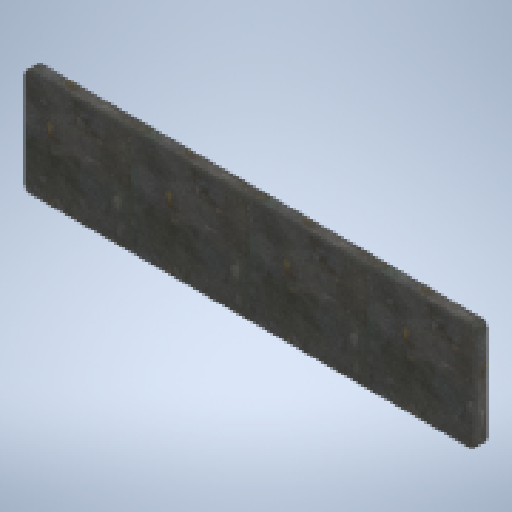
# Autodesk Inventor part: MountingPlate
Saved by Autodesk Inventor 2023 (Build 270158000, 158)
## iProperties
Created: 2023-07-27
Part Number: MountingPlate
Material: Steel
Document SubType Name: Modeling
Designer: Parker
Density: 7.85 g/cm^3
Appearance: Plate
Author: Parker
Autodesk Inventor part; units mm, degrees
ref_plane "YZ Plane" through (0, 0, 0) normal (1, 0, 0) x (0, 1, 0)
ref_plane "XZ Plane" through (0, 0, 0) normal (0, 1, 0) x (-1, 0, 0)
ref_plane "XY Plane" through (0, 0, 0) normal (0, 0, 1) x (1, 0, 0)
sketch "Sketch1" plane through (0, 0, 0) normal (0, 0, 1) x (1, 0, 0)
  circle A0 centre (323.7, 80.7) radius 3.75 projected
  circle A1 centre (224.8, -20.2) radius 3.75 projected
  line L0 (219.8, -29.2) -> (328.7, -29.2) projected
  arc A2 (215.8, -25.2) -> (219.8, -29.2) centre (219.8, -25.2) ccw projected
  line L1 (215.8, 85.7) -> (215.8, -25.2) projected
  arc A3 (219.8, 89.7) -> (215.8, 85.7) centre (219.8, 85.7) ccw projected
  line L2 (328.7, 89.7) -> (219.8, 89.7) projected
  arc A4 (332.7, 85.7) -> (328.7, 89.7) centre (328.7, 85.7) ccw projected
  line L3 (332.7, -25.2) -> (332.7, 85.7) projected
  arc A5 (328.7, -29.2) -> (332.7, -25.2) centre (328.7, -25.2) ccw projected
  circle A6 centre (224.8, 80.7) radius 3.75 projected
  circle A7 centre (323.7, -20.2) radius 3.75 projected
  circle A8 centre (-229.1, -19.7) radius 3.75 projected
  circle A9 centre (-288.2, -19.7) radius 3.75 projected
  circle A10 centre (-170, 80.7) radius 3.75 projected
  line L4 (-165, 89.7) -> (-293.2, 89.7) projected
  arc A11 (-161, 85.7) -> (-165, 89.7) centre (-165, 85.7) ccw projected
  line L5 (-161, -24.7) -> (-161, 85.7) projected
  arc A12 (-165, -28.7) -> (-161, -24.7) centre (-165, -24.7) ccw projected
  line L6 (-293.2, -28.7) -> (-165, -28.7) projected
  arc A13 (-297.2, -24.7) -> (-293.2, -28.7) centre (-293.2, -24.7) ccw projected
  line L7 (-297.2, 85.7) -> (-297.2, -24.7) projected
  arc A14 (-293.2, 89.7) -> (-297.2, 85.7) centre (-293.2, 85.7) ccw projected
  circle A15 centre (-170, -19.7) radius 3.75 projected
  circle A16 centre (-288.2, 80.7) radius 3.75 projected
  circle A17 centre (-229.1, 80.7) radius 3.75 projected
  line L8 (352.7, 109.7) -> (-317.2, 109.7)
  line L9 (-317.2, 109.7) -> (-317.2, -49.2)
  line L10 (-317.2, -49.2) -> (352.7, -49.2)
  line L11 (352.7, -49.2) -> (352.7, 109.7)
  point P0 (0, 0)
  dimension "d0" = 20
  dimension "d1" = 20
  dimension "d2" = 20
  dimension "d3" = 20
  constraints: 8 end point, 2 parallel, 1 horizontal, 1 perpendicular
  measures "d0" distance between parallel lines of L2 L8
  measures "d1" distance between parallel lines of L3 L11
  measures "d2" distance between parallel lines of L10 L0
  measures "d3" distance between parallel lines of L7 L9
extrude "Extrusion1" add sketch "Sketch1" against normal blind 20 contours A0 | A1 | A2 L1 A3 L2 A4 L3 A5 L0 | A6 | A7 | A8 | A9 | A10 | A11 L5 A12 L6 A13 L7 A14 L4 | A15 | A16 | A17 | L11 L10 L9 L8
fillet "Fillet1" radius 10 4 edges at (352.7, 109.7, -10) (352.7, -49.2, -10) (-317.2, -49.2, -10) (-317.2, 109.7, -10)
sketch "Sketch2" plane through (0, 0, 0) normal (0, 0, 1) x (1, 0, 0)
  circle A0 centre (323.7, -20.2) radius 2.75 projected
  circle A1 centre (224.8, -20.2) radius 2.75 projected
  circle A2 centre (323.7, 80.7) radius 3.75 projected
  circle A3 centre (224.8, 80.7) radius 3.75 projected
  circle A4 centre (-170, 80.7) radius 3.75 projected
  circle A5 centre (-229.1, 80.7) radius 3.75 projected
  circle A6 centre (-288.2, 80.7) radius 3.75 projected
  circle A7 centre (-288.2, -19.7) radius 2.75 projected
  circle A8 centre (-229.1, -19.7) radius 2.75 projected
  circle A9 centre (-170, -19.7) radius 3.75 projected
  point P0 (0, 0)
hole "Hole1" at (323.7, 80.7, 0) at (224.8, 80.7, 0) at (323.7, -20.2, 0) at (224.8, -20.2, 0) at (-170, -19.7, 0) at (-229.1, -19.7, 0) at (-288.2, -19.7, 0) at (-288.2, 80.7, 0) at (-229.1, 80.7, 0) at (-170, 80.7, 0) direction (0, 0, -1) diameter 4.134 end through all thread size "M5x0.8" class "6H" standard "ANSI Metric M Profile"
chamfer "Chamfer1" distance 2 angle 45 10 edges at (323.7, -18.133, 0) (323.7, 82.767, 0) (224.8, 82.767, 0) (224.8, -18.133, 0) (-170, -17.633, 0) (-170, 82.767, 0) (-229.1, 82.767, 0) (-288.2, 82.767, 0) (-288.2, -17.633, 0) (-229.1, -17.633, 0)
chamfer "Chamfer2" distance 2 angle 45 16 edges at (17.75, 109.7, 0) (-314.2711, 106.7711, 0) (-317.2, 30.25, 0) (-314.2711, -46.2711, 0) (17.75, -49.2, 0) (349.7711, -46.2711, 0) (352.7, 30.25, 0) (349.7711, 106.7711, 0) (17.75, 109.7, -20) (349.7711, 106.7711, -20) (352.7, 30.25, -20) (349.7711, -46.2711, -20) (17.75, -49.2, -20) (-314.2711, -46.2711, -20) (-317.2, 30.25, -20) (-314.2711, 106.7711, -20)
body "Solid1"
